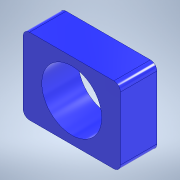
# Autodesk Inventor part: Gearbox Mount
Saved by Autodesk Inventor 2022 (Build 260153000, 153)
## iProperties
Created: 2022-08-13
Part Number: Gearbox Mount
Material: Generic
Document SubType Name: Modeling
Designer: Nick
Density: 0.513495 g/cm^3
Appearance: Blue - Wall Paint - Glossy
Mass: 20 g
Surface Area: 107.38 cm^2
Volume: 38.9487 cm^3
Author: Nick
Autodesk Inventor part; units mm, degrees
ref_plane "YZ Plane" through (0, 0, 0) normal (1, 0, 0) x (0, 1, 0)
ref_plane "XZ Plane" through (0, 0, 0) normal (0, 1, 0) x (-1, 0, 0)
ref_plane "XY Plane" through (0, 0, 0) normal (0, 0, 1) x (1, 0, 0)
sketch "Sketch1" plane through (0, 0, 0) normal (0, 0, 1) x (1, 0, 0)
  line L0 (0, 0) -> (60, 0)
  line L1 (60, 0) -> (60, 47)
  line L2 (60, 47) -> (0, 47)
  line L3 (0, 47) -> (0, 0)
  circle A0 centre (30, 23.5) radius 18.5
  line L4 (11.5, 42) -> (48.5, 42) construction
  line L5 (48.5, 42) -> (48.5, 5) construction
  line L6 (48.5, 5) -> (11.5, 5) construction
  line L7 (11.5, 5) -> (11.5, 42) construction
  point P0 (60, 23.5)
  point P1 (30, 47)
  dimension "d0" = 37
  dimension "d1" = 5
  dimension "d5" = 60
  constraints: 16 end point, 4 parallel, 4 tangent, 2 horizontal, 2 midpoint, 2 perpendicular, 1 centre point, 1 horizontal alignment, 1 vertical alignment
  measures "d0" diameter of A0
  measures "d1" distance between parallel lines of L2 L4
  measures "d5" distance of L1.end L2.end
extrude "Extrusion1" add sketch "Sketch1" along normal blind 22.5
fillet "Fillet1" radius 4 4 edges at (60, 47, 11.25) (60, 0, 11.25) (0, 0, 11.25) (0, 47, 11.25)
body "Solid1"
